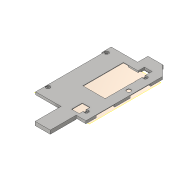
# Autodesk Inventor part: 01_Adapter
Saved by Autodesk Inventor 2016 (Build 200138000, 138)
## iProperties
Created: 2017-04-20
Part Number: 01_Adapter
Material: Generisch
Document SubType Name: Modeling
Designer: diederichbenedict
Density: 1 g/cm^3
Appearance: Vorgabe
Mass: 5.2527 g
Surface Area: 54.5277 cm^2
Volume: 5.2527 cm^3
Author: diederichbenedict
Autodesk Inventor part; units mm, degrees
ref_plane "YZ Plane" through (0, 0, 0) normal (1, 0, 0) x (0, 1, 0)
ref_plane "XZ Plane" through (0, 0, 0) normal (0, 1, 0) x (-1, 0, 0)
ref_plane "XY Plane" through (0, 0, 0) normal (0, 0, 1) x (1, 0, 0)
ref_plane "Arbeitsebene1" through (0, 0, 0) normal (0, 0, 1) x (1, 0, 0)
sketch "Skizze1" plane through (0, 0, 0) normal (0, 0, 1) x (1, 0, 0)
  line L0 (17.0472, 13) -> (17.0472, -9.5) construction
  line L1 (17.0472, -9.5) -> (13.0472, -9.5) construction
  line L2 (13.0472, -9.5) -> (13.0472, -23.5) construction
  line L3 (13.0472, -23.5) -> (-13.9528, -23.5) construction
  line L4 (-13.9528, -23.5) -> (-13.9528, 31.5) construction
  line L5 (-13.9528, 31.5) -> (-20.9528, 31.5) construction
  line L6 (-20.9528, 31.5) -> (-20.9528, -31.5) construction
  line L7 (-20.9528, -31.5) -> (23.0472, -31.5) construction
  arc A0 (23.0472, -31.5) -> (23.0472, 31.5) centre (-98.984, 0) ccw construction
  line L8 (23.0472, 31.5) -> (17.0472, 31.5) construction
  line L9 (17.0472, 31.5) -> (17.0472, 23) construction
  line L10 (17.0472, 23) -> (17.0472, 13) construction
  circle A1 centre (-17.9528, -27) radius 1 projected
  circle A2 centre (23.0472, 9) radius 1 construction
  circle A3 centre (21.0472, 28) radius 1 projected
  circle A4 centre (-18.4528, 30) radius 1 projected
  circle A5 centre (21.0472, -29) radius 1 projected
  circle A6 centre (-17.9528, -8) radius 1 projected
  line L11 (7.0472, 13) -> (17.0472, 13) construction
  line L12 (17.0472, 13) -> (17.0472, 23) construction
  line L13 (17.0472, 23) -> (7.0472, 23) construction
  line L14 (7.0472, 23) -> (7.0472, 13) construction
  circle A7 centre (12.0472, 18) radius 7.5
  line L15 (7.0472, 23) -> (17.0472, 23) projected
  line L16 (17.0472, 23) -> (17.0472, 31.5) projected
  line L17 (17.0472, 31.5) -> (-13.9528, 31.5) projected
  line L18 (-13.9528, 31.5) -> (-13.9528, -23.5) projected
  line L19 (-13.9528, -23.5) -> (13.0472, -23.5) projected
  line L20 (13.0472, -23.5) -> (13.0472, -9.5) projected
  line L21 (13.0472, -9.5) -> (17.0472, -9.5) projected
  line L22 (17.0472, -9.5) -> (17.0472, 13) projected
  line L23 (17.0472, 13) -> (7.0472, 13) projected
  line L24 (7.0472, 13) -> (7.0472, 23) projected
  line L25 (19.5472, 37) -> (19.5472, 23)
  line L26 (19.5472, 23) -> (25.5472, 23)
  line L27 (25.5472, 23) -> (25.5472, 13)
  line L28 (25.5472, 13) -> (19.5472, 13)
  line L29 (19.5472, 13) -> (19.5472, 3)
  line L30 (19.5472, 3) -> (25.5472, 3)
  line L31 (25.5472, 3) -> (25.5472, -27)
  line L32 (25.5472, -27) -> (19.5472, -27)
  line L33 (19.5472, -27) -> (19.5472, -33)
  line L34 (19.5472, -33) -> (28.5472, -33)
  line L35 (28.5472, 37) -> (19.5472, 37)
  line L36 (-20.9528, 28) -> (-14.9528, 28)
  line L37 (-14.9528, 28) -> (-14.9528, 37)
  line L38 (-14.9528, 37) -> (-20.9528, 37)
  line L39 (-20.9528, 37) -> (-20.9528, 28)
  line L40 (19.5472, 37) -> (-14.9528, 37)
  line L41 (-14.9528, 37) -> (-14.9528, 33)
  line L42 (-14.9528, 33) -> (19.5472, 33)
  line L43 (19.5472, 33) -> (19.5472, 37)
  line L44 (-19.9528, -33) -> (-14.9528, -33)
  line L45 (-14.9528, -33) -> (-14.9528, -24)
  line L46 (-14.9528, -24) -> (-19.9528, -24)
  line L47 (-19.9528, -24) -> (-19.9528, -33)
  line L48 (28.5472, -33) -> (-19.9528, -33)
  line L49 (-19.9528, -33) -> (-19.9528, -37)
  line L50 (-19.9528, -37) -> (28.5472, -37)
  line L51 (28.5472, 37) -> (4.5472, 37)
  line L52 (28.5472, 37) -> (28.5472, -37)
  circle A8 centre (24.0472, 9) radius 1
  point P0 (0, 0)
  dimension "d0" = 15
  dimension "d1" = 10
  dimension "d2" = 30
  dimension "d3" = 6
  dimension "d7" = 6
  dimension "d8" = 4
  dimension "d9" = 5
  dimension "d10" = 9
  dimension "d11" = 34.5
  dimension "d12" = 4
  dimension "d52" = 7.5
  dimension "d75" = 2
  dimension "d76" = 1
  dimension "d87" = 3
  dimension "d88" = 0
  constraints: 56 end point, 9 perpendicular, 9 point on line, 7 parallel, 5 horizontal, 2 centre point, 2 vertical
  measures "d0" diameter of A7
  measures "d1" distance of L28.end L29.end
  measures "d2" distance of L30.end L31.end
  measures "d3" distance of L32.end L33.end
  measures "d7" distance of L38.end L37.end
  measures "d8" distance of L41.end L40.end
  measures "d9" distance of L46.end L45.end
  measures "d10" distance of L45.end L44.end
  measures "d11" distance between parallel lines of L45 L33
  measures "d12" distance of L49.end L48.end
  measures "d52" distance from line of L52 A5.centre
  measures "d75" diameter of A8
  measures "d76" distance of A8.centre A2.centre
  measures "d87" distance between parallel lines of L31 L52
  measures "d88" distance between parallel lines of L26 L13
extrude "Extrusion1" add sketch "Skizze1" along normal blind 1 contours L35 L52 L34 L33 L32 L31 L30 L29 L28 L27 L26 L25 | L25 L42 L37 L40 | L37 L36 L39 L38 | L52 L50 L49 L44 L48 L34 | L44 L47 L46 L45
sketch "Skizze2" plane through (0, 0, 1) normal (0, 0, 1) x (1, 0, 0)
  circle A0 centre (21.0472, -29) radius 1 projected
  circle A1 centre (21.0472, 28) radius 1 projected
  circle A2 centre (-18.4528, 30) radius 1 projected
  circle A3 centre (-17.9528, -27) radius 1 projected
  line L0 (-14.9528, -33) -> (-14.9528, -24) projected
  line L1 (-14.9528, -24) -> (-19.9528, -24) projected
  line L2 (-19.9528, -24) -> (-19.9528, -37) projected
  line L3 (-19.9528, -37) -> (28.5472, -37) projected
  line L4 (-20.9528, 37) -> (-20.9528, 28) projected
  line L5 (-20.9528, 28) -> (-14.9528, 28) projected
  line L6 (-14.9528, 28) -> (-14.9528, 33) projected
  line L7 (-14.9528, 33) -> (19.5472, 33) projected
  line L8 (19.5472, 33) -> (19.5472, 23) projected
  line L9 (19.5472, 23) -> (25.5472, 23) projected
  line L10 (25.5472, 23) -> (25.5472, 13) projected
  line L11 (25.5472, 13) -> (19.5472, 13) projected
  line L12 (19.5472, 13) -> (19.5472, 3) projected
  line L13 (19.5472, 3) -> (25.5472, 3) projected
  line L14 (25.5472, 3) -> (25.5472, -27) projected
  line L15 (25.5472, -27) -> (19.5472, -27) projected
  line L16 (19.5472, -27) -> (19.5472, -33) projected
  line L17 (19.5472, -33) -> (-14.9528, -33) projected
  circle A4 centre (21.0472, 28) radius 1
  circle A5 centre (24.0472, 9) radius 1
  circle A6 centre (21.0472, -29) radius 1
  circle A7 centre (-17.9528, -27) radius 1
  circle A8 centre (-18.4528, 30) radius 1
  line L18 (28.5472, 37) -> (-20.9528, 37) projected
  line L19 (28.5472, -37) -> (28.5472, 37) projected
  circle A9 centre (24.0472, 9) radius 1 projected
  point P0 (0, 0)
  dimension "d15" = 0
  dimension "d17" = 0
  dimension "d18" = 0
  dimension "d19" = 0
  constraints: 5 centre point, 1 coincident
  measures "d15" radial gap between concentric circles of A1 A4
  measures "d17" radial gap between concentric circles of A0 A6
  measures "d18" radial gap between concentric circles of A3 A7
  measures "d19" radial gap between concentric circles of A2 A8
extrude "Extrusion2" add sketch "Skizze2" along normal blind 1
sketch "Skizze3" plane through (0, 0, 2) normal (0, 0, 1) x (1, 0, 0)
  line L0 (7.0472, 13) -> (17.0472, 13) projected
  line L1 (17.0472, 13) -> (17.0472, 23) projected
  line L2 (17.0472, 23) -> (7.0472, 23) projected
  line L3 (7.0472, 23) -> (7.0472, 13) projected
  circle A0 centre (12.0472, 18) radius 7.5
  circle A1 centre (-18.4528, 30) radius 1 projected
  circle A2 centre (-17.9528, -27) radius 1 projected
  line L4 (-14.9528, -33) -> (-14.9528, -24) projected
  line L5 (-14.9528, -24) -> (-19.9528, -24) projected
  line L6 (-19.9528, -24) -> (-19.9528, -37) projected
  line L7 (-19.9528, -37) -> (28.5472, -37) projected
  line L8 (-20.9528, 37) -> (-20.9528, 28) projected
  line L9 (-20.9528, 28) -> (-14.9528, 28) projected
  line L10 (-14.9528, 28) -> (-14.9528, 33) projected
  line L11 (-14.9528, 33) -> (19.5472, 33) projected
  line L12 (19.5472, 33) -> (19.5472, 23) projected
  circle A3 centre (21.0472, 28) radius 1 projected
  line L13 (19.5472, 23) -> (25.5472, 23) projected
  line L14 (25.5472, 23) -> (25.5472, 13) projected
  line L15 (25.5472, 13) -> (19.5472, 13) projected
  line L16 (19.5472, 13) -> (19.5472, 3) projected
  line L17 (19.5472, 3) -> (25.5472, 3) projected
  line L18 (25.5472, 3) -> (25.5472, -27) projected
  line L19 (25.5472, -27) -> (19.5472, -27) projected
  line L20 (19.5472, -27) -> (19.5472, -33) projected
  circle A4 centre (21.0472, -29) radius 1 projected
  line L21 (19.5472, -33) -> (-14.9528, -33) projected
  circle A5 centre (24.0472, 9) radius 1 projected
  line L22 (19.5472, 33) -> (2.5472, 33)
  line L23 (2.5472, 33) -> (2.5472, 3)
  line L24 (2.5472, 3) -> (19.5472, 3)
  line L25 (19.5472, 3) -> (19.5472, 33)
  line L26 (25.5472, 23) -> (19.5472, 23)
  line L27 (19.5472, 23) -> (19.5472, 13)
  line L28 (19.5472, 13) -> (25.5472, 13)
  line L29 (25.5472, 13) -> (25.5472, 23)
  line L30 (28.5472, 37) -> (-20.9528, 37) projected
  line L31 (28.5472, -37) -> (28.5472, 37) projected
  point P0 (0, 0)
  dimension "d22" = 15
  dimension "d23" = 17
  constraints: 16 end point, 4 parallel, 2 horizontal, 2 perpendicular, 1 centre point
  measures "d22" diameter of A0
  measures "d23" distance of L24.end L23.end
extrude "Extrusion3" add sketch "Skizze3" along normal blind 1 contours L25 L13 L14 L15 | L25 L16 L24 L23 L11 L12 | L15 L14 L13 L12 L11 L10 L9 L8 L30 L31 L7 L6 L5 L4 L21 L20 L19 L18 L17 L16
sketch "Skizze12" plane through (0, 0, 0) normal (0, 0, -1) x (-1, 0, 0)
  circle A0 centre (-21.0472, -29) radius 1 projected
  circle A1 centre (-21.0472, 28) radius 1 projected
  circle A2 centre (17.9528, -27) radius 1 projected
  circle A3 centre (18.4528, 30) radius 1 projected
  line L0 (20.9528, 28) -> (14.9528, 28) projected
  line L1 (20.9528, 37) -> (20.9528, 28) projected
  line L2 (-28.5472, 37) -> (20.9528, 37) projected
  line L3 (-28.5472, -37) -> (-28.5472, 37) projected
  line L4 (19.9528, -37) -> (-28.5472, -37) projected
  line L5 (19.9528, -24) -> (19.9528, -37) projected
  line L6 (14.9528, -24) -> (19.9528, -24) projected
  line L7 (14.9528, -33) -> (14.9528, -24) projected
  line L8 (-19.5472, -33) -> (14.9528, -33) projected
  line L9 (-19.5472, -27) -> (-19.5472, -33) projected
  line L10 (-25.5472, -27) -> (-19.5472, -27) projected
  line L11 (-25.5472, 3) -> (-25.5472, -27) projected
  line L12 (-19.5472, 3) -> (-25.5472, 3) projected
  line L13 (-19.5472, 13) -> (-19.5472, 3) projected
  line L14 (-25.5472, 13) -> (-19.5472, 13) projected
  line L15 (-25.5472, 23) -> (-25.5472, 13) projected
  line L16 (-19.5472, 23) -> (-25.5472, 23) projected
  line L17 (-19.5472, 33) -> (-19.5472, 23) projected
  line L18 (14.9528, 33) -> (-19.5472, 33) projected
  line L19 (14.9528, 28) -> (14.9528, 33) projected
  line L20 (-28.5472, -37) -> (-28.5472, 37) projected
  line L21 (-19.5472, -33) -> (14.9528, -33) projected
  line L22 (-28.5472, 33) -> (-19.5472, 33)
  line L23 (-19.5472, 33) -> (-19.5472, -33)
  line L24 (-19.5472, -33) -> (-28.5472, -33)
  line L25 (-28.5472, -33) -> (-28.5472, 33)
  point P0 (0, 0)
  constraints: 8 end point, 2 parallel, 1 horizontal, 1 perpendicular, 1 point on line
extrude "Extrusion10" cut sketch "Skizze12" against normal blind 1 contours L17 L16 L15 L14 L13 L12 L11 L10 L9 L24 L3 L22 | L23 L14 L15 L16 | L23 L10 L11 L12
sketch "Skizze13" plane through (0, 0, 3) normal (0, 0, 1) x (1, 0, 0)
  line L0 (19.5472, 23) -> (25.5472, 23) projected
  circle A0 centre (24.0472, 9) radius 1 projected
  line L1 (2.5472, 3) -> (25.5472, 3) projected
  line L2 (25.5472, 3) -> (25.5472, -27) projected
  line L3 (25.5472, -27) -> (19.5472, -27) projected
  line L4 (19.5472, -27) -> (19.5472, -33) projected
  circle A1 centre (21.0472, -29) radius 1 projected
  line L5 (19.5472, -33) -> (-14.9528, -33) projected
  line L6 (-14.9528, -33) -> (-14.9528, -24) projected
  line L7 (-14.9528, -24) -> (-19.9528, -24) projected
  line L8 (-19.9528, -24) -> (-19.9528, -37) projected
  line L9 (-19.9528, -37) -> (28.5472, -37) projected
  line L10 (28.5472, -37) -> (28.5472, 37) projected
  line L11 (28.5472, 37) -> (-20.9528, 37) projected
  line L12 (-20.9528, 37) -> (-20.9528, 28) projected
  line L13 (-20.9528, 28) -> (-14.9528, 28) projected
  line L14 (-14.9528, 28) -> (-14.9528, 33) projected
  line L15 (-14.9528, 33) -> (2.5472, 33) projected
  line L16 (2.5472, 33) -> (2.5472, 3) projected
  circle A2 centre (12.0472, 18) radius 7.5 projected
  circle A3 centre (-18.4528, 30) radius 1 projected
  circle A4 centre (-17.9528, -27) radius 1 projected
  circle A5 centre (21.0472, 28) radius 1 projected
  line L17 (28.5472, 37) -> (-20.9528, 37) projected
  line L18 (-19.9528, -37) -> (28.5472, -37) projected
  line L19 (19.5472, 37) -> (-5.4528, 37)
  line L20 (-5.4528, 37) -> (-5.4528, -37)
  line L21 (-5.4528, -37) -> (19.5472, -37)
  line L22 (19.5472, -37) -> (19.5472, 37)
  line L23 (25.5472, 3) -> (25.5472, -27) projected
  circle A6 centre (21.0472, -29) radius 1 projected
  line L24 (25.5472, -27) -> (19.5472, -27) projected
  line L25 (19.5472, 13) -> (19.5472, 3) projected
  line L26 (19.5472, -27) -> (25.5472, -27)
  line L27 (25.5472, -27) -> (25.5472, 3)
  line L28 (25.5472, 3) -> (19.5472, 3)
  line L29 (19.5472, 3) -> (19.5472, -27)
  line L30 (-19.9528, -37) -> (-5.4528, -37)
  line L31 (-5.4528, -37) -> (-5.4528, 37)
  line L32 (-5.4528, 37) -> (-19.9528, 37)
  line L33 (-19.9528, 37) -> (-19.9528, -37)
  point P0 (0, 0)
  point P1 (19.5472, -29)
  dimension "d55" = 25
  constraints: 24 end point, 6 parallel, 3 horizontal, 3 perpendicular, 2 coincident, 2 horizontal alignment, 2 point on line
  measures "d55" distance of L21.end L20.end
extrude "Extrusion11" add sketch "Skizze13" along normal blind 0.5
sketch "Skizze16" plane through (0, 0, 3.5) normal (0, 0, 1) x (1, 0, 0)
  circle A0 centre (12.0472, 18) radius 7.5 projected
  line L0 (4.5472, 18) -> (19.1472, 18)
  line L1 (19.1472, 18) -> (19.1472, -62)
  line L2 (19.1472, -62) -> (4.5472, -62)
  line L3 (4.5472, -62) -> (4.5472, 18)
  line L4 (-19.9528, -37) -> (28.5472, -37) projected
  line L5 (4.5472, -37) -> (19.1472, -37)
  line L6 (19.1472, -37) -> (19.1472, -62)
  line L7 (19.1472, -62) -> (4.5472, -62)
  line L8 (4.5472, -62) -> (4.5472, -37)
  line L9 (28.5472, 37) -> (-20.9528, 37) projected
  line L10 (4.5472, 37) -> (19.1472, 37)
  line L11 (19.1472, 37) -> (19.1472, 47)
  line L12 (19.1472, 47) -> (4.5472, 47)
  line L13 (4.5472, 47) -> (4.5472, 37)
  line L14 (19.1472, -12.1185) -> (19.1472, 28.8815) projected
  point P0 (0, 0)
  dimension "d60" = 80
  dimension "d61" = 10
  dimension "d68" = 0
  constraints: 24 end point, 7 point on line, 6 parallel, 3 horizontal, 3 perpendicular, 1 horizontal alignment, 1 other
  measures "d60" distance of L0.end L1.end
  measures "d61" distance of L11.end L10.end
  measures "d68" distance between parallel lines of L1 L14
extrude "Extrusion12" add sketch "Skizze16" against normal up to surface (3.5 mm away) contours L4 L1 L2 L3 | L9 L13 L12 L11
sketch "Skizze18" plane through (0, 0, 3.5) normal (0, 0, 1) x (1, 0, 0)
  line L0 (12.1472, -24) -> (19.1472, -24) projected
  line L1 (19.1472, -24) -> (19.1472, -34) projected
  line L2 (19.1472, -34) -> (12.1472, -34) projected
  line L3 (12.1472, -34) -> (12.1472, -24) projected
  line L4 (12.1472, 1) -> (19.1472, 1) construction
  line L5 (19.1472, 1) -> (19.1472, -9) construction
  line L6 (19.1472, -9) -> (12.1472, -9) construction
  line L7 (12.1472, -9) -> (12.1472, 1) construction
  line L8 (12.1472, 1) -> (19.1472, 1) construction
  line L9 (19.1472, 1) -> (19.1472, -9) construction
  line L10 (19.1472, -9) -> (12.1472, -9) construction
  line L11 (12.1472, -9) -> (12.1472, 1) construction
  line L12 (19.3472, -23.8) -> (11.9472, -23.8)
  line L13 (11.9472, -23.8) -> (11.9472, -34.2)
  line L14 (11.9472, -34.2) -> (19.3472, -34.2)
  line L15 (19.3472, -34.2) -> (19.3472, -23.8)
  line L16 (12.1472, -9) -> (19.1472, -9) construction
  line L17 (19.1472, -9) -> (19.1472, 1) construction
  line L18 (19.1472, 1) -> (12.1472, 1) construction
  line L19 (12.1472, 1) -> (12.1472, -9) construction
  line L20 (19.1472, -9) -> (12.1472, -9)
  line L21 (12.1472, -9) -> (12.1472, 1)
  line L22 (12.1472, 1) -> (19.1472, 1)
  line L23 (19.1472, 1) -> (19.1472, -9)
  line L24 (11.9472, -9.2) -> (19.3472, -9.2)
  line L25 (19.3472, -9.2) -> (19.3472, 1.2)
  line L26 (19.3472, 1.2) -> (11.9472, 1.2)
  line L27 (11.9472, 1.2) -> (11.9472, -9.2)
  line L28 (19.1472, 36) -> (12.1472, 36) projected
  line L29 (12.1472, 26) -> (19.1472, 26) projected
  line L30 (19.1472, 36) -> (12.1472, 36)
  line L31 (12.1472, 36) -> (12.1472, 26)
  line L32 (12.1472, 26) -> (19.1472, 26)
  line L33 (19.1472, 26) -> (19.1472, 36)
  line L34 (11.9472, 25.8) -> (11.9472, 36.2)
  line L35 (11.9472, 36.2) -> (19.3472, 36.2)
  line L36 (19.3472, 36.2) -> (19.3472, 25.8)
  line L37 (19.3472, 25.8) -> (11.9472, 25.8)
  point P0 (0, 0)
  dimension "d69" = 0.2
  dimension "d70" = 0.2
  dimension "d71" = 0.2
  dimension "d84" = 0.2
  dimension "d85" = 0.2
  dimension "d86" = 0.2
  constraints: 48 end point, 10 parallel, 5 perpendicular, 4 horizontal, 6 other
  measures "d69" distance between parallel lines of L0 L12
  measures "d70" distance between parallel lines of L4 L26
  measures "d71" distance between parallel lines of L5 L25
  measures "d84" distance between parallel lines of L31 L34
  measures "d85" distance between parallel lines of L16 L24
  measures "d86" distance between parallel lines of L7 L27
extrude "Extrusion14" cut sketch "Skizze18" against normal through all contours L0 L1 L2 L3 | L15 L14 L13 L12 | L20 L21 L22 L23 | L27 L26 L25 L24 | L33 L29 L31 L28 | L34 L35 L36 L37
sketch "Skizze17" plane through (0, 0, 0) normal (0, 0, -1) x (-1, 0, 0)
  circle A0 centre (18.4528, 30) radius 1 projected
  line L0 (14.9528, 33) -> (-11.9472, 33) projected
  line L1 (14.9528, 28) -> (14.9528, 33) projected
  line L2 (20.9528, 28) -> (14.9528, 28) projected
  line L3 (20.9528, 37) -> (20.9528, 28) projected
  line L4 (-4.5472, 37) -> (20.9528, 37) projected
  line L5 (-4.5472, 47) -> (-4.5472, 37) projected
  line L6 (-19.1472, 47) -> (-4.5472, 47) projected
  line L7 (-19.1472, 37) -> (-19.1472, 47) projected
  line L8 (-28.5472, 37) -> (-19.1472, 37) projected
  line L9 (-28.5472, 33) -> (-28.5472, 37) projected
  circle A1 centre (17.9528, -27) radius 1 projected
  line L10 (-28.5472, -33) -> (-19.3472, -33) projected
  line L11 (-28.5472, -37) -> (-28.5472, -33) projected
  line L12 (-19.1472, -37) -> (-28.5472, -37) projected
  line L13 (-19.1472, -62) -> (-19.1472, -37) projected
  line L14 (-4.5472, -62) -> (-19.1472, -62) projected
  line L15 (-4.5472, -37) -> (-4.5472, -62) projected
  line L16 (19.9528, -37) -> (-4.5472, -37) projected
  line L17 (19.9528, -24) -> (19.9528, -37) projected
  line L18 (14.9528, -24) -> (19.9528, -24) projected
  line L19 (14.9528, -33) -> (14.9528, -24) projected
  circle A2 centre (-12.0472, 42) radius 4.1
  circle A3 centre (-12.0472, -56) radius 4.1
  line L20 (-11.9472, -33) -> (-11.9472, -34.2) projected
  line L21 (-11.9472, -34.2) -> (-19.3472, -34.2) projected
  line L22 (-19.3472, -34.2) -> (-19.3472, -33) projected
  line L23 (-11.9472, -33) -> (14.9528, -33) projected
  line L24 (-11.9472, -33) -> (-11.9472, -34.2) projected
  line L25 (-11.9472, -34.2) -> (-19.3472, -34.2) projected
  line L26 (-19.3472, -34.2) -> (-19.3472, -33) projected
  line L27 (-19.1472, -37) -> (-28.5472, -37) projected
  line L28 (-19.1472, -62) -> (-19.1472, -37) projected
  line L29 (-4.5472, -62) -> (-19.1472, -62) projected
  line L30 (-4.5472, -37) -> (-4.5472, -62) projected
  line L31 (19.9528, -37) -> (-4.5472, -37) projected
  line L32 (19.9528, -24) -> (19.9528, -37) projected
  line L33 (14.9528, -24) -> (19.9528, -24) projected
  line L34 (14.9528, -33) -> (14.9528, -24) projected
  line L35 (14.9528, 28) -> (14.9528, 33) projected
  line L36 (20.9528, 28) -> (14.9528, 28) projected
  line L37 (20.9528, 37) -> (20.9528, 28) projected
  line L38 (-4.5472, 37) -> (20.9528, 37) projected
  line L39 (-4.5472, 47) -> (-4.5472, 37) projected
  line L40 (-19.1472, 47) -> (-4.5472, 47) projected
  line L41 (-19.1472, 37) -> (-19.1472, 47) projected
  line L42 (-28.5472, 37) -> (-19.1472, 37) projected
  line L43 (-28.5472, -33) -> (-19.3472, -33) projected
  line L44 (-28.5472, -37) -> (-28.5472, -33) projected
  line L45 (-11.9472, -33) -> (14.9528, -33) projected
  line L46 (14.9528, 33) -> (-11.9472, 33) projected
  line L47 (-28.5472, 33) -> (-28.5472, 37) projected
  line L48 (-11.9472, 36.2) -> (-11.9472, 33) projected
  line L49 (-19.3472, 33) -> (-28.5472, 33) projected
  line L50 (-19.3472, 33) -> (-19.3472, 36.2) projected
  line L51 (-19.3472, 36.2) -> (-11.9472, 36.2) projected
  line L52 (-11.9472, 36.2) -> (-11.9472, 33) projected
  line L53 (-19.3472, 33) -> (-28.5472, 33) projected
  line L54 (-19.3472, 33) -> (-19.3472, 36.2) projected
  line L55 (-19.3472, 36.2) -> (-11.9472, 36.2) projected
  point P0 (0, 0)
  dimension "d64" = 8.2
  dimension "d65" = 8.2
  dimension "d74" = 6
  constraints: 2 centre point
  measures "d64" diameter of A2
  measures "d65" diameter of A3
  measures "d74" distance from line of A3.centre L14
extrude "Extrusion13" cut sketch "Skizze17" against normal blind 3 contours A2 | A3
sketch "Skizze19" plane through (0, 0, 3.5) normal (0, 0, 1) x (1, 0, 0)
  line L0 (11.9472, -34.2) -> (11.9472, -23.8) projected
  line L1 (11.9472, -23.8) -> (19.3472, -23.8) projected
  line L2 (19.3472, -23.8) -> (19.3472, -34.2) projected
  line L3 (19.3472, -34.2) -> (11.9472, -34.2) projected
  line L4 (19.3472, 1.2) -> (19.3472, -9.2) projected
  line L5 (19.3472, -9.2) -> (11.9472, -9.2) projected
  line L6 (11.9472, -9.2) -> (11.9472, 1.2) projected
  line L7 (11.9472, 1.2) -> (19.3472, 1.2) projected
  circle A0 centre (-17.9528, -27) radius 1 projected
  circle A1 centre (12.0472, 18) radius 7.5 projected
  circle A2 centre (-18.4528, 30) radius 1 projected
  circle A3 centre (21.0472, 28) radius 1 projected
  circle A4 centre (21.0472, -29) radius 1 projected
  circle A5 centre (24.0472, 9) radius 1 projected
  line L8 (-19.9528, -37) -> (4.5472, -37) projected
  line L9 (4.5472, -37) -> (4.5472, -62) projected
  line L10 (4.5472, -62) -> (19.1472, -62) projected
  line L11 (19.1472, -62) -> (19.1472, -37) projected
  line L12 (19.1472, -37) -> (28.5472, -37) projected
  line L13 (28.5472, -37) -> (28.5472, 37) projected
  line L14 (28.5472, 37) -> (19.1472, 37) projected
  line L15 (19.1472, 37) -> (19.1472, 47) projected
  line L16 (19.1472, 47) -> (4.5472, 47) projected
  line L17 (4.5472, 47) -> (4.5472, 37) projected
  line L18 (4.5472, 37) -> (-20.9528, 37) projected
  line L19 (-20.9528, 37) -> (-20.9528, 28) projected
  line L20 (-20.9528, 28) -> (-19.9528, 28) projected
  line L21 (-19.9528, 28) -> (-19.9528, -37) projected
  circle A6 centre (-17.9528, -27) radius 2
  circle A7 centre (21.0472, -29) radius 2
  circle A8 centre (24.0472, 9) radius 2
  circle A9 centre (21.0472, 28) radius 2
  circle A10 centre (-18.4528, 30) radius 2
  point P0 (0, 0)
  dimension "d77" = 1
  dimension "d78" = 1
  dimension "d79" = 1
  dimension "d80" = 1
  dimension "d81" = 1
  constraints: 5 centre point
  measures "d77" radial gap between concentric circles of A0 A6
  measures "d78" radial gap between concentric circles of A4 A7
  measures "d79" radial gap between concentric circles of A5 A8
  measures "d80" radial gap between concentric circles of A3 A9
  measures "d81" radial gap between concentric circles of A2 A10
extrude "Extrusion15" cut sketch "Skizze19" against normal blind 1 contours A7 L2 | L2 A7 | A6 | A8 | A9 | A10
sketch "Skizze21" plane through (0, 0, 0) normal (0, 0, -1) x (-1, 0, 0)
  circle A0 centre (-12.0472, -56) radius 4.1 projected
  circle A1 centre (17.9528, -27) radius 1 projected
  line L0 (-11.9472, -33) -> (-11.9472, -34.2) projected
  line L1 (-11.9472, -34.2) -> (-19.3472, -34.2) projected
  line L2 (-19.3472, -34.2) -> (-19.3472, -33) projected
  line L3 (-28.5472, -33) -> (-19.3472, -33) projected
  line L4 (-28.5472, -37) -> (-28.5472, -33) projected
  line L5 (-19.1472, -37) -> (-28.5472, -37) projected
  line L6 (-19.1472, -62) -> (-19.1472, -37) projected
  line L7 (-4.5472, -62) -> (-19.1472, -62) projected
  line L8 (-4.5472, -37) -> (-4.5472, -62) projected
  line L9 (19.9528, -37) -> (-4.5472, -37) projected
  line L10 (19.9528, -24) -> (19.9528, -37) projected
  line L11 (14.9528, -24) -> (19.9528, -24) projected
  line L12 (14.9528, -33) -> (14.9528, -24) projected
  line L13 (-11.9472, -33) -> (14.9528, -33) projected
  circle A2 centre (-12.0472, 42) radius 4.1 projected
  line L14 (-11.9472, 36.2) -> (-11.9472, 33) projected
  line L15 (14.9528, 33) -> (-11.9472, 33) projected
  line L16 (14.9528, 28) -> (14.9528, 33) projected
  line L17 (20.9528, 28) -> (14.9528, 28) projected
  line L18 (20.9528, 37) -> (20.9528, 28) projected
  line L19 (-4.5472, 37) -> (20.9528, 37) projected
  line L20 (-4.5472, 47) -> (-4.5472, 37) projected
  line L21 (-19.1472, 47) -> (-4.5472, 47) projected
  line L22 (-19.1472, 37) -> (-19.1472, 47) projected
  line L23 (-28.5472, 37) -> (-19.1472, 37) projected
  line L24 (-28.5472, 33) -> (-28.5472, 37) projected
  line L25 (-19.3472, 33) -> (-28.5472, 33) projected
  line L26 (-19.3472, 33) -> (-19.3472, 36.2) projected
  line L27 (-19.3472, 36.2) -> (-11.9472, 36.2) projected
  circle A3 centre (18.4528, 30) radius 1 projected
  line L28 (-28.5472, -37) -> (20.9528, -37)
  line L29 (20.9528, -37) -> (20.9528, 37)
  line L30 (20.9528, 37) -> (-28.5472, 37)
  line L31 (-28.5472, 37) -> (-28.5472, -37)
  point P0 (0, 0)
  constraints: 8 end point, 2 parallel, 1 horizontal, 1 perpendicular
extrude "Extrusion16" cut sketch "Skizze21" against normal up to surface (1 mm away) contours L13 L12 L11 L10 L9 L28 L5 L4 L3 L2 L1 L0 | L0 L1 L2 L3 L31 L25 L26 L27 L14 L15 L16 L17 L29 L28 L10 L11 L12 L13 | L24 L23 L30 L19 L18 L17 L16 L15 L14 L27 L26 L25
sketch "Skizze22" plane through (0, 0, 1) normal (0, 0, -1) x (-1, 0, 0)
  circle A0 centre (18.4528, 30) radius 1 projected
  circle A1 centre (17.9528, -27) radius 1 projected
  circle A2 centre (-21.0472, -29) radius 1 projected
  circle A3 centre (-21.0472, 28) radius 1 projected
  circle A4 centre (-24.0472, 9) radius 1 projected
  line L0 (-19.5472, 3) -> (-25.5472, 3) projected
  line L1 (-19.5472, 13) -> (-19.5472, 3) projected
  line L2 (-25.5472, 13) -> (-19.5472, 13) projected
  line L3 (-25.5472, 23) -> (-25.5472, 13) projected
  line L4 (-19.5472, 23) -> (-25.5472, 23) projected
  line L5 (-19.5472, 33) -> (-19.5472, 23) projected
  line L6 (-19.3472, 33) -> (-19.5472, 33) projected
  line L7 (-19.3472, 36.2) -> (-19.3472, 33) projected
  line L8 (-11.9472, 36.2) -> (-19.3472, 36.2) projected
  line L9 (-11.9472, 33) -> (-11.9472, 36.2) projected
  line L10 (14.9528, 33) -> (-11.9472, 33) projected
  line L11 (14.9528, 28) -> (14.9528, 33) projected
  line L12 (20.9528, 28) -> (14.9528, 28) projected
  line L13 (20.9528, 37) -> (20.9528, 28) projected
  line L14 (-4.5472, 37) -> (20.9528, 37) projected
  line L15 (-4.5472, 37) -> (-19.1472, 37) projected
  line L16 (-28.5472, 37) -> (-19.1472, 37) projected
  line L17 (-28.5472, -37) -> (-28.5472, 37) projected
  line L18 (-19.1472, -37) -> (-28.5472, -37) projected
  line L19 (-19.1472, -37) -> (-4.5472, -37) projected
  line L20 (19.9528, -37) -> (-4.5472, -37) projected
  line L21 (19.9528, -24) -> (19.9528, -37) projected
  line L22 (14.9528, -24) -> (19.9528, -24) projected
  line L23 (14.9528, -33) -> (14.9528, -24) projected
  line L24 (-11.9472, -33) -> (14.9528, -33) projected
  line L25 (-11.9472, -34.2) -> (-11.9472, -33) projected
  line L26 (-19.3472, -34.2) -> (-11.9472, -34.2) projected
  line L27 (-19.3472, -33) -> (-19.3472, -34.2) projected
  line L28 (-19.5472, -33) -> (-19.3472, -33) projected
  line L29 (-19.5472, -27) -> (-19.5472, -33) projected
  line L30 (-25.5472, -27) -> (-19.5472, -27) projected
  line L31 (-25.5472, 3) -> (-25.5472, -27) projected
  line L32 (-28.5472, -37) -> (-28.5472, 37) projected
  line L33 (-19.5472, -27) -> (-28.5472, -27)
  line L34 (-28.5472, -27) -> (-28.5472, -9)
  line L35 (-28.5472, -9) -> (-19.5472, -9)
  line L36 (-19.5472, -9) -> (-19.5472, -27)
  point P0 (0, 0)
  dimension "d91" = 18
  constraints: 8 end point, 2 parallel, 1 horizontal, 1 perpendicular, 1 point on line
  measures "d91" distance of L33.end L34.end
extrude "Extrusion17" cut sketch "Skizze22" against normal up to surface (2 mm away) contours L35 L36 L30 L31 | L31 L33 L17 L35
chamfer "Fase1" distance 9.4 angle 45 1 edges at (19.1472, 37, 2.25)
sketch "Skizze23" plane through (0, 0, 3.5) normal (0, 0, 1) x (1, 0, 0)
  circle A0 centre (-18.4528, 30) radius 2 projected
  circle A1 centre (24.0472, 9) radius 2 projected
  circle A2 centre (-17.9528, -27) radius 2 projected
  arc A3 (19.3472, -30.0536) -> (19.3472, -27.9464) centre (21.0472, -29) ccw projected
  arc A4 (19.3472, 26.9464) -> (19.3472, 29.0536) centre (21.0472, 28) ccw projected
  line L0 (19.3472, 1.2) -> (19.3472, -9.2) projected
  line L1 (19.3472, -9.2) -> (11.9472, -9.2) projected
  line L2 (11.9472, -9.2) -> (11.9472, 1.2) projected
  line L3 (11.9472, 1.2) -> (19.3472, 1.2) projected
  line L4 (11.9472, -34.2) -> (11.9472, -23.8) projected
  line L5 (11.9472, -23.8) -> (19.3472, -23.8) projected
  line L6 (19.3472, -30.0536) -> (19.3472, -34.2) projected
  line L7 (19.3472, -34.2) -> (11.9472, -34.2) projected
  line L8 (19.3472, 25.8) -> (11.9472, 25.8) projected
  line L9 (11.9472, 25.8) -> (11.9472, 36.2) projected
  line L10 (11.9472, 36.2) -> (19.3472, 36.2) projected
  line L11 (19.3472, 26.9464) -> (19.3472, 25.8) projected
  line L12 (-19.9528, 28) -> (-19.9528, -27) projected
  line L13 (-19.9528, -37) -> (4.5472, -37) projected
  line L14 (4.5472, -37) -> (4.5472, -62) projected
  line L15 (4.5472, -62) -> (19.1472, -62) projected
  line L16 (19.1472, -62) -> (19.1472, -37) projected
  line L17 (19.1472, -37) -> (28.5472, -37) projected
  line L18 (28.5472, -37) -> (28.5472, 37) projected
  line L19 (19.1472, 46.4) -> (28.5472, 37) projected
  line L20 (19.1472, 46.4) -> (19.1472, 47) projected
  line L21 (19.1472, 47) -> (4.5472, 47) projected
  line L22 (4.5472, 47) -> (4.5472, 37) projected
  line L23 (4.5472, 37) -> (-20.9528, 37) projected
  line L24 (-20.9528, 37) -> (-20.9528, 28) projected
  line L25 (-20.9528, 28) -> (-19.9528, 28) projected
  circle A5 centre (12.0472, 18) radius 7.5 projected
  line L26 (19.3472, -9.2) -> (11.9472, -9.2) projected
  line L27 (19.3472, -9.2) -> (-2.1766, -9.2)
  line L28 (-2.1766, -9.2) -> (-2.1766, 30)
  line L29 (-2.1766, 30) -> (19.3472, 30)
  line L30 (19.3472, 30) -> (19.3472, -9.2)
  line L31 (-19.9528, -27) -> (-19.9528, -37) projected
  line L32 (19.3472, 36.2) -> (19.3472, 29.0536) projected
  line L33 (19.3472, -23.8) -> (19.3472, -27.9464) projected
  point P0 (0, 0)
  constraints: 8 end point, 2 parallel, 1 horizontal, 1 horizontal alignment, 1 perpendicular
extrude "Extrusion18" cut sketch "Skizze23" against normal blind 10 contours L11 L8 L9 L29 L30 | L30 A5 L3 L2 L27 L28 L29 L9 L8 | L30 A5 picked at (15.1128, 18.5735)
sketch "Skizze24" plane through (28.5472, -37, 1) normal (1, 0, 0) x (0, 0, -1)
  line L0 (-2, 28) -> (0, 28) projected
  line L1 (0, 28) -> (0, 74) projected
  line L2 (0, 74) -> (-2.5, 74) projected
  line L3 (-2.5, 0) -> (-2.5, 74) projected
  line L4 (0, 0) -> (-2.5, 0) projected
  line L5 (0, 0) -> (0, 10) projected
  line L6 (0, 10) -> (-2, 10) projected
  line L7 (-2, 10) -> (-2, 28) projected
  line L8 (-2, 65) -> (-2, 13) projected
  line L9 (0, 62.6632) -> (-2, 62.6632)
  line L10 (-2, 62.6632) -> (-2, 42.6632)
  line L11 (-2, 42.6632) -> (0, 42.6632)
  line L12 (0, 42.6632) -> (0, 62.6632)
  point P0 (1, 37)
  dimension "d99" = 20
  constraints: 8 end point, 2 parallel, 2 point on line, 1 horizontal, 1 perpendicular
  measures "d99" distance of L10.end L9.end
extrude "Extrusion19" cut sketch "Skizze24" against normal blind 10 contours L8 L9 L1 L11
